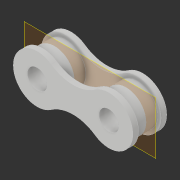
# Autodesk Inventor part: Inner Chain
Saved by Autodesk Inventor 2019 (Build 230136000, 136)
## iProperties
Created: 2020-06-03
Part Number: Inner Chain
Material: Generic
Document SubType Name: Modeling
Designer: 18186
Density: 1 g/cm^3
Appearance: Default
Author: 18186
Autodesk Inventor part; units mm, degrees
ref_plane "YZ Plane" through (0, 0, 0) normal (1, 0, 0) x (0, 1, 0)
ref_plane "XZ Plane" through (0, 0, 0) normal (0, 1, 0) x (-1, 0, 0)
ref_plane "XY Plane" through (0, 0, 0) normal (0, 0, 1) x (1, 0, 0)
sketch "Sketch1" plane through (0, 0, 0) normal (0, 0, 1) x (1, 0, 0)
  arc A0 (-3.9144, 3.4829) -> (-3.9144, -3.4829) centre (-6.35, 0) ccw
  arc A1 (3.9144, -3.4829) -> (3.9144, 3.4829) centre (6.35, 0) ccw
  line L0 (0, 0) -> (0, 6.6345) construction
  circle A2 centre (-6.35, 0) radius 3.6195
  line L1 (-6.35, -4.25) -> (6.35, -4.25) construction
  arc A3 (3.9144, -3.4829) -> (-3.9144, -3.4829) centre (0, -9.0806) ccw
  arc A4 (-3.9144, 3.4829) -> (3.9144, 3.4829) centre (0, 9.0806) ccw
  circle A5 centre (6.35, 0) radius 3.6195
  circle A6 centre (-6.35, 0) radius 1.75
  circle A7 centre (6.35, 0) radius 1.75
  point P0 (0, -2.25)
  point P1 (0, 2.25)
  point P2 (0, -2.25)
  dimension "d0" = 12.7
  dimension "d1" = 8.5
  dimension "d2" = 8.5
  dimension "d3" = 7.239
  dimension "d5" = 4.5
  dimension "d6" = 7.239
  dimension "d7" = 3.5
  dimension "d8" = 3.5
  constraints: 12 point on circle, 8 centre point, 5 coincident, 4 end point, 3 horizontal alignment, 3 tangent, 2 vertical alignment, 1 symmetric about line, 1 vertical
  measures "d0" distance of A1.centre A0.centre
  measures "d1" diameter of A0
  measures "d2" diameter of A1
  measures "d3" diameter of A2
  measures "d5" distance of point (0, -2.25) point (0, 2.25)
  measures "d6" diameter of A5
  measures "d7" diameter of A6
  measures "d8" diameter of A7
extrude "Extrusion1" add sketch "Sketch1" against normal blind 1 contours A4 A1 A3 A0 | A2 | A5
extrude "Extrusion2" add sketch "Sketch1" along normal blind 4 contours A2 | A5
ref_plane "Work Plane1" through (0, 0, 2) normal (0, 0, 1) x (1, 0, 0)
mirror "Mirror1" about plane through (0, 0, 2) normal (0, 0, 1) of "Extrusion1"
ref_plane "Work Plane2" through (0, 9.0806, 2) normal (0, 0, 1) x (1, 0, 0)
equation "\"d2\" = d1"
equation "\"d6\" = d3"
equation "\"d7\" = d8"
body "Solid1"
